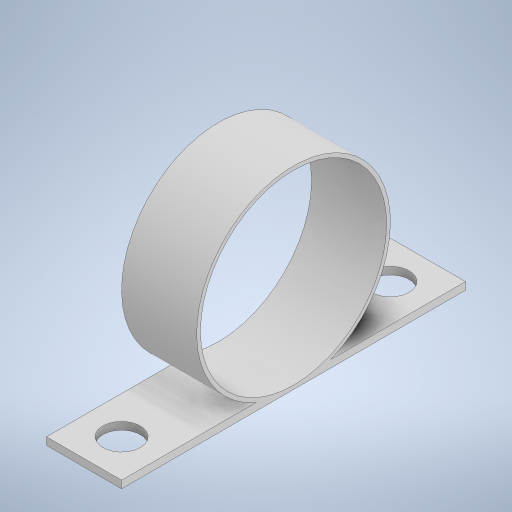
# Autodesk Inventor part: apoiom
Saved by Autodesk Inventor 2024 (Build 280153020, 153B)
## iProperties
Created: 2023-06-05
Part Number: apoiom
Material: Genérico
Document SubType Name: Modeling
Designer: victo
Density: 1 g/cm^3
Appearance: Padrão
Author: victo
Autodesk Inventor part; units mm, degrees
ref_plane "YZ Plane" through (0, 0, 0) normal (1, 0, 0) x (0, 1, 0)
ref_plane "XZ Plane" through (0, 0, 0) normal (0, 1, 0) x (-1, 0, 0)
ref_plane "XY Plane" through (0, 0, 0) normal (0, 0, 1) x (1, 0, 0)
sketch "Esboço1" plane through (0, 0, 0) normal (1, 0, 0) x (0, 1, 0)
  arc A0 (-11.9, -4.98) -> (-11.9, 4.98) centre (0, 0) ccw
  circle A1 centre (0, 0) radius 12.4
  line L0 (-12.9, 0) -> (-12.9, -10)
  line L1 (-12.9, -10) -> (-12.9, -12.9)
  line L2 (-12.9, -12.9) -> (-12.9, -22.9)
  line L3 (-12.9, -22.9) -> (-11.9, -22.9)
  line L4 (-11.9, -22.9) -> (-11.9, -4.98)
  line L5 (-12.9, 0) -> (-12.9, 22.9)
  line L6 (-12.9, 22.9) -> (-11.9, 22.9)
  line L7 (-11.9, 22.9) -> (-11.9, 4.98)
  dimension "d57" = 25.8
  dimension "d58" = 24.8
  dimension "d59" = 10
  dimension "d60" = 10
  dimension "d61" = 1
  dimension "d62" = 22.9
  dimension "d63" = 1
  constraints: 16 end point, 4 point on line, 2 centre point, 2 perpendicular, 2 point on circle, 2 vertical, 1 coincident, 1 tangent
  measures "d57" diameter of A0
  measures "d58" diameter of A1
  measures "d59" distance of L0.start L0.end
  measures "d60" distance of L1.end L2.end
  measures "d61" distance of L2.end L3.end
  measures "d62" distance of L0.start L5.end
  measures "d63" distance of L5.end L6.end
extrude "Extrusão6" add sketch "Esboço1" against normal blind 10
sketch "Esboço6" plane through (0, -11.9, -4.98) normal (0, 1, 0) x (1, 0, 0)
  line L0 (0, 17.92) -> (-10, 17.92) projected
  line L1 (0, -27.88) -> (-10, -27.88) projected
  circle A0 centre (-5, -22.88) radius 2.5
  circle A1 centre (-5, 12.92) radius 2.5
  point P0 (0, -4.98)
  dimension "d68" = 5
  dimension "d69" = 5
  constraints: 2 centre point
  measures "d68" diameter of A0
  measures "d69" diameter of A1
extrude "Extrusão7" cut sketch "Esboço6" against normal up to next
